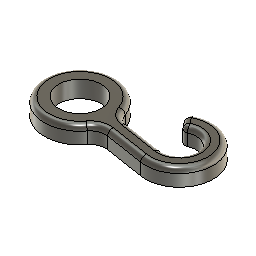
Hook (Autodesk Fusion 360 design; units mm, degrees)
Autodesk Fusion 360 part; units mm, degrees
sketch "Sketch2" plane through (0, 0, 0) normal (0, 0, 1) x (1, 0, 0)
  circle A0 centre (-15.2715, 3.416) radius 25
  circle A1 centre (-15.2715, 3.416) radius 42
  line L0 (26.2114, -3.1542) -> (83.4973, -12.2274)
  line L1 (-15.2715, 3.416) -> (54.7285, 3.416) construction
  arc A2 (83.4973, -12.2274) -> (69.6032, 40.9514) centre (88.1903, 17.4032) ccw
  dimension "d1" = 50
  dimension "d2" = 84
  dimension "d3" = 100
  dimension "d4" = 9
  dimension "d5" = 30
  constraint concentric A0 A1
  constraint horizontal L1
  constraint coincident A0.centre A1.centre
  constraint tangent L0 A2
  constraint coincident A1 L0.start
  measures "d1" diameter of A0
  measures "d2" diameter of A1
  measures "d3" distance of A0.centre L0.end
  measures "d4" angle of L0 L1
  measures "d5" radius of A2
extrude "Extrude1" add sketch "Sketch2" along normal blind 20 makes body 1
surface "Extrude2" add extruded along (0, 0, 1) between 0 and 20 path "Sketch2" along L0 A2 separate body makes body 2
thicken "Thicken1" add thickness 10 on both sides 2 faces at (64.402, -9.203, 6.6667) (70.7782, 41.8331, 6.6667) separate body on bodies 2 makes body 3
extrude "Extrude3" add 1 faces at (26.7328, 0.1381, 13.3333) along direction (-0.987688, 0.156434, 0) blind 2 on bodies 3 bodies 3 1
fillet "Fillet2" radius 6 2 edges at (75.7989, 33.102, 10) (63.4075, 48.8008, 10) on bodies 3
fillet "Fillet3" radius 18 2 edges at (23.454, -12.8422, 10) (26.5827, 6.9116, 10) on bodies 3
fillet "Fillet4" radius 6 10 edges at (25.9916, -15.862, 20) (58.7549, -18.4333, 20) (127.6348, 24.0466, 20) (66.2919, 48.6165, 20) (69.9859, 40.4666, 20) (75.8368, 35.1412, 20) (107.9971, 20.1767, 20) (61.8836, 1.3205, 20) (29.9292, 8.9995, 20) (-56.7545, 9.9863, 20) on bodies 3
hidden bodies 2
equation "d18 = FRad"
equation "d20 = FRad * 3"
equation "d22 = FRad"
equation "FRad = 6 mm"
